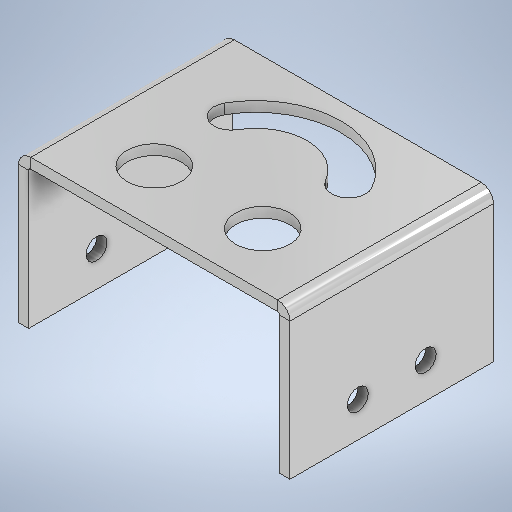
# Autodesk Inventor part: Head2
Saved by Autodesk Inventor 2026.1 (Build 301233000, 233)
## iProperties
Created: 2025-08-16
Part Number: Head2
Material: Aluminum 6061-AHC
Document SubType Name: Sheet Metal
Designer: chris
Density: 2.7 g/cm^3
Sheet Metal Rule: Default_mm
Appearance: Aluminum - Dark
Flat Pattern Width: 3 cm
Flat Pattern Length: 7.85586 cm
Flat Pattern Area: 23.5676 cm^2
Sheet Metal Width: 30.000 mm
Sheet Metal Length: 78.559 mm
Sheet Metal Area: 2356.757 mm^2
Author: chris
Autodesk Inventor part; units mm, degrees
ref_plane "YZ Plane" through (0, 0, 0) normal (1, 0, 0) x (0, 1, 0)
ref_plane "XZ Plane" through (0, 0, 0) normal (0, 1, 0) x (-1, 0, 0)
ref_plane "XY Plane" through (0, 0, 0) normal (0, 0, 1) x (1, 0, 0)
sketch "Sketch1" plane through (0, 0, 0) normal (0, 1, 0) x (-1, 0, 0)
  line L0 (20, -15) -> (-20, -15)
  line L1 (-20, -15) -> (-20, 15)
  line L2 (-20, 15) -> (20, 15)
  line L3 (20, 15) -> (20, -15)
  line L4 (20, -15) -> (-20, 15) construction
  line L5 (-20, -15) -> (20, 15) construction
  point P0 (0, 0)
  dimension "d0" = 40
  dimension "d1" = 30
  measures "d0" distance of L1.end L2.end
  measures "d1" distance of L0.end L1.end
extrude "Plate1" add sketch "Sketch1" along normal blind 1.5
sketch "Sketch2" plane through (18.5, 1.5, 15) normal (1, 0, 0) x (0, 1, 0)
  line L0 (0, -30) -> (0, 0)
  line L1 (0, 0) -> (-22, 0)
  line L2 (-22, 0) -> (-22, -30)
  line L3 (-22, -30) -> (0, -30)
  constraints: 6 end point, 1 horizontal, 1 perpendicular, 1 vertical
edge flange "Flange1" height 22 angle 90 thickness 1.5 bend radius 0.31 thickness toward (1, 0, 0) relief tear relief width 1.5 relief depth 0.75 corner gap 0.31 corner form 0 edges at (20, 0, 0) (-20, 0, 0) wall of the first edge with corners at (18.5, 1.5, -15) (18.5, 1.5, 15) (18.5, -20.5, 15) (18.5, -20.5, -15)
bend "Bend1"
corner "Corner1"
sketch "Sketch3" plane through (20, -20.5, 15) normal (1, 0, 0) x (0, 0, -1)
  circle A0 centre (20, 5.19) radius 1.55
  circle A1 centre (10, 5.19) radius 1.55
  line L0 (30, 20.19) -> (0, 20.19) projected
  line L1 (30, 0) -> (30, 20.19) projected
  point P0 (15, 20.5)
  dimension "d13" = 3.1
  dimension "d14" = 3.1
  dimension "d15" = 15
  dimension "d16" = 15
  dimension "d17" = 10
  dimension "d33" = 10
  constraints: 2 centre point
  measures "d13" diameter of A0
  measures "d14" diameter of A1
  measures "d15" distance from line of A1.centre L0
  measures "d16" distance from line of L0 A0.centre
  measures "d17" distance of A0.centre A1.centre
  measures "d33" distance from line of L1 A0.centre
extrude "Cut1" cut sketch "Sketch3" against normal through all
sketch "Sketch4" plane through (0, 1.5, 0) normal (0, 1, 0) x (1, 0, 0)
  circle A0 centre (8, -7) radius 4
  circle A1 centre (-8, -7) radius 4
  arc A2 (0, 10) -> (-8.6603, 5) centre (0, 0) ccw construction
  arc A3 (0, 12.5) -> (-10.8253, 6.25) centre (0, 0) ccw
  arc A4 (0, 7.5) -> (-6.4952, 3.75) centre (0, 0) ccw
  arc A5 (0, 7.5) -> (0, 12.5) centre (0, 10) ccw
  arc A6 (-10.8253, 6.25) -> (-6.4952, 3.75) centre (-8.6603, 5) ccw
  line L0 (0, 0) -> (-8.6603, 5) construction
  line L1 (0, 0) -> (0, 10) construction
  arc A7 (8.6603, 5) -> (0, 10) centre (0, 0) ccw construction
  arc A8 (10.8253, 6.25) -> (0, 12.5) centre (0, 0) ccw
  arc A9 (6.4952, 3.75) -> (0, 7.5) centre (0, 0) ccw
  arc A10 (6.4952, 3.75) -> (10.8253, 6.25) centre (8.6603, 5) ccw
  arc A11 (0, 12.5) -> (0, 7.5) centre (0, 10) ccw
  line L2 (0, 0) -> (8.6603, 5) construction
  line L3 (0, 0) -> (0, 10) construction
  dimension "d20" = 8
  dimension "d21" = 8
  dimension "d22" = 10
  dimension "d23" = 60
  dimension "d24" = 5
  dimension "d25" = 60
  dimension "d26" = 5
  dimension "d27" = 7
  dimension "d28" = 7
  dimension "d29" = 8
  dimension "d30" = 8
  constraints: 20 point on circle, 12 centre point, 8 end point, 8 tangent, 2 coincident
  measures "d20" diameter of A0
  measures "d21" diameter of A1
  measures "d22" radius of A2
  measures "d23" angle of L1 L0
  measures "d24" diameter of A6
  measures "d25" angle of L2 L3
  measures "d26" diameter of A10
  measures "d27" vertical distance of point (0, 0) A1.centre
  measures "d28" vertical distance of A0.centre point (0, 0)
  measures "d29" horizontal distance of point (0, 0) A1.centre
  measures "d30" horizontal distance of A0.centre point (0, 0)
extrude "Cut2" cut sketch "Sketch4" against normal through all
equation "\"d16\" = d15"
equation "\"d18\" = Thickness"
equation "\"d28\" = d27"
equation "\"d30\" = d29"
equation "\"d31\" = Thickness"
equation "\"d2\" = Thickness"
equation "\"d3\" = BendReliefWidth"
equation "\"d4\" = BendReliefDepth"
equation "\"d5\" = MinimumRemnant"
equation "\"d6\" = TransitionRadius"
equation "\"d9\" = BendRadius"
equation "\"d10\" = CornerReliefSize"
equation "\"d11\" = GapSize"
equation "\"d12\" = JacobiRadiusSize"
equation "\"BendReliefWidth\" = Thickness"
equation "\"BendReliefDepth\" = 0.5 * Thickness"
equation "\"CornerReliefSize\" = 4 * Thickness"
equation "\"MinimumRemnant\" = 2 * Thickness"
equation "\"TransitionRadius\" = BendRadius"
equation "\"JacobiRadiusSize\" = BendRadius"
equation "\"GapSize\" = Thickness"
equation "\"Thickness\" = 1.5"
equation "\"BendRadius\" = 0.31"
body "Solid1"
